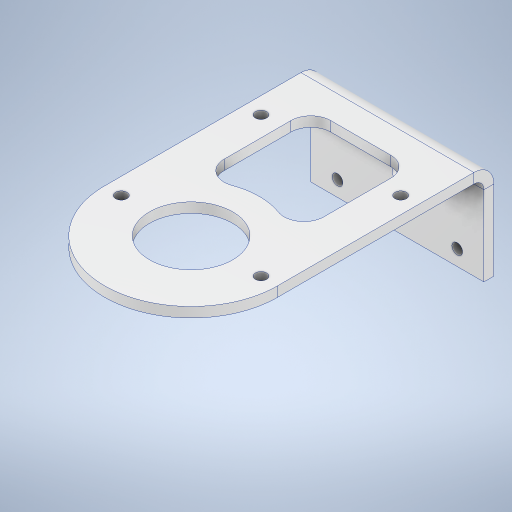
# Autodesk Inventor part: toe_front
Saved by Autodesk Inventor 2024.1 (Build 281209000, 209)
## iProperties
Created: 2024-02-12
Part Number: toe_front
Material: アルミニウム 6061
Document SubType Name: Sheet Metal
Designer: hibik
Density: 2.7 g/cm^3
Sheet Metal Rule: Default_mm
Appearance: アルミニウム - フラット
Flat Pattern Width: 2.6 cm
Flat Pattern Length: 5.78929 cm
Flat Pattern Area: 15.0522 cm^2
Sheet Metal Width: 26.000 mm
Sheet Metal Length: 57.893 mm
Sheet Metal Area: 1505.216 mm^2
Author: hibik
Autodesk Inventor part; units mm, degrees
ref_plane "YZ Plane" through (0, 0, 0) normal (1, 0, 0) x (0, 1, 0)
ref_plane "XZ Plane" through (0, 0, 0) normal (0, 1, 0) x (-1, 0, 0)
ref_plane "XY Plane" through (0, 0, 0) normal (0, 0, 1) x (1, 0, 0)
sketch "スケッチ1" plane through (0, 0, 0) normal (0, 1, 0) x (-1, 0, 0)
  line L0 (26, 0) -> (0, 0)
  line L1 (0, 0) -> (0, -89.5474)
  line L2 (0, -89.5474) -> (26, -89.5474)
  line L3 (26, -89.5474) -> (26, 0)
  line L4 (26, 0) -> (0, 0)
  line L5 (0, 0) -> (0, 70)
  line L6 (0, 70) -> (26, 70)
  line L7 (26, 70) -> (26, 0)
  line L8 (26, 32.5) -> (0, 32.5)
  circle A0 centre (13, 32.5) radius 6.25
  circle A1 centre (13, 32.5) radius 13
  point P0 (26, 32.5)
  point P1 (0, 32.5)
  dimension "d2" = 70
  dimension "d3" = 26
  dimension "d4" = 32.5
  dimension "d5" = 12.5
  measures "d2" distance of L4.end L5.end
  measures "d3" distance of L5.end L6.end
  measures "d4" distance between parallel lines of L0 L8
  measures "d5" diameter of A0
extrude "プレート1" add sketch "スケッチ1" along normal blind 1.5 contours L0 L5 A1 L7 | A1 L8 A0 | L8 A0 A1
sketch "スケッチ3" plane through (0, 1.5, 0) normal (0, 1, 0) x (1, 0, 0)
  circle A0 centre (-23.5, -32.5) radius 0.85 projected
  circle A1 centre (-23.5, -11.5) radius 0.85 projected
  circle A2 centre (-2.5, -11.5) radius 0.85 projected
  circle A3 centre (-2.5, -32.5) radius 0.85 projected
  point P0 (0, 0)
extrude "切り取り1" cut sketch "スケッチ3" against normal blind 1.5
sketch "スケッチ4" plane through (0, 1.5, 1.5) normal (0, 0, -1) x (-1, 0, 0)
  line L0 (26, 0) -> (0, 0)
  line L1 (0, 0) -> (0, -15)
  line L2 (0, -15) -> (26, -15)
  line L3 (26, -15) -> (26, 0)
  constraints: 6 end point, 1 horizontal, 1 perpendicular, 1 vertical
edge flange "フランジ2" height 15 angle 90 thickness 1.5 bend radius 1.5 thickness toward (0, 0, -1) relief straight relief width 1.5 relief depth 0.75 edges at (-13, 0, 0) wall of the first edge with corners at (-26, 1.5, 1.5) (0, 1.5, 1.5) (0, -13.5, 1.5) (-26, -13.5, 1.5)
bend "曲げ2"
corner "コーナー2"
sketch "スケッチ5" plane through (0, -13.5, 0) normal (0, 0, -1) x (-1, 0, 0)
  line L0 (0, 0) -> (26, 0)
  line L1 (26, 0) -> (26, 15)
  line L2 (26, 15) -> (0, 15)
  line L3 (0, 15) -> (0, 0)
  line L4 (26, 12) -> (26, 0) projected
  line L5 (0, 0) -> (0, 12) projected
  line L6 (0, 15) -> (26, 0)
  line L7 (26, 15) -> (0, 0)
  line L8 (4, 12.6923) -> (22, 12.6923)
  line L9 (22, 12.6923) -> (22, 2.3077)
  line L10 (22, 2.3077) -> (4, 2.3077)
  line L11 (4, 2.3077) -> (4, 12.6923)
  circle A0 centre (4, 12.6923) radius 0.8
  circle A1 centre (22, 12.6923) radius 0.8
  circle A2 centre (4, 2.3077) radius 0.8
  circle A3 centre (22, 2.3077) radius 0.8
  circle A4 centre (13, 7.5) radius 0.8
  point P0 (0, 13.5)
  dimension "d35" = 15
  dimension "d36" = 4
  dimension "d37" = 1.6
  dimension "d38" = 1.6
  dimension "d39" = 1.6
  dimension "d40" = 1.6
  dimension "d43" = 1.6
  constraints: 20 end point, 5 centre point, 4 coincident, 4 parallel, 3 point on line, 2 collinear, 2 horizontal, 2 perpendicular, 1 midpoint
  measures "d35" distance between parallel lines of L0 L2
  measures "d36" distance between parallel lines of L3 L11
  measures "d37" diameter of A0
  measures "d38" diameter of A1
  measures "d39" diameter of A2
  measures "d40" diameter of A3
  measures "d43" diameter of A4
extrude "切り取り3" cut sketch "スケッチ5" against normal blind 1.5 contours A2 L11 L7 | L7 L10 A2 | A3 L10 L6 | L6 L9 A3 | L11 A2 L7 | L7 A2 L10 | L10 A3 L6 | L6 A3 L9 | A4 L6 L7 | L7 L6 A4 | L6 L7 A4 | L6 A4 L7
sketch "スケッチ6" plane through (0, 1.5, 0) normal (0, 1, 0) x (1, 0, 0)
  circle A0 centre (-2.5, -32.5) radius 0.85 projected
  circle A1 centre (-23.5, -32.5) radius 0.85 projected
  circle A2 centre (-23.5, -11.5) radius 0.85 projected
  circle A3 centre (-2.5, -11.5) radius 0.85 projected
  line L0 (-2.5, -32.5) -> (-23.5, -32.5)
  line L1 (-23.5, -32.5) -> (-23.5, -11.5)
  line L2 (-23.5, -11.5) -> (-2.5, -11.5)
  line L3 (-2.5, -11.5) -> (-2.5, -32.5)
  line L4 (-5.5, -32.5) -> (-20.5, -32.5)
  line L5 (-20.5, -20.0376) -> (-20.5, -10)
  line L6 (-17.5, -7) -> (-8.5, -7)
  line L7 (-5.5, -10) -> (-5.5, -20.0376)
  circle A4 centre (-13, -32.5) radius 6.25 projected
  line L8 (0, -3) -> (-26, -3) projected
  arc A5 (-9.5189, -22.8592) -> (-16.4811, -22.8592) centre (-13, -32.5) ccw
  arc A6 (-23.2186, -31.6979) -> (-23.2186, -33.3021) centre (-13, -32.5) ccw
  arc A7 (-2.7814, -33.3021) -> (-2.7814, -31.6979) centre (-13, -32.5) ccw
  arc A8 (-9.5189, -22.8592) -> (-5.5, -20.0376) centre (-8.5, -20.0376) ccw
  arc A9 (-20.5, -20.0376) -> (-16.4811, -22.8592) centre (-17.5, -20.0376) ccw
  arc A10 (-5.5, -10) -> (-8.5, -7) centre (-8.5, -10) ccw
  arc A11 (-17.5, -7) -> (-20.5, -10) centre (-17.5, -10) ccw
  point P0 (0, 0)
  point P1 (-20.5, -7)
  point P2 (-5.5, -7)
  point P3 (-5.5, -25.5134)
  point P4 (-20.5, -25.5134)
  dimension "d46" = 3
  dimension "d47" = 3
  dimension "d49" = 4
  dimension "d50" = 4
  dimension "d53" = 3
  dimension "d54" = 3
  constraints: 20 point on circle, 16 end point, 8 tangent, 7 centre point, 7 point on line, 4 parallel, 2 equal radius, 2 horizontal, 2 perpendicular, 1 concentric, 1 midpoint
  measures "d46" distance between parallel lines of L3 L7
  measures "d47" distance between parallel lines of L1 L5
  measures "d49" distance between parallel lines of L8 L6
  measures "d50" radial gap between concentric circles of A4 A5
  measures "d53" radius of A8
  measures "d54" radius of A9
extrude "切り取り4" cut sketch "スケッチ6" against normal blind 1.5 contours L7 A8 A5 A9 L5 L2 | L2 L5 A11 L6 A10 L7
equation "\"d23\" = Thickness"
equation "\"d44\" = Thickness"
equation "\"d51\" = Thickness"
equation "\"d12\" = Thickness"
equation "\"d25\" = BendReliefWidth"
equation "\"d26\" = BendReliefDepth"
equation "\"d27\" = MinimumRemnant"
equation "\"d28\" = TransitionRadius"
equation "\"d31\" = BendRadius"
equation "\"d32\" = CornerReliefSize"
equation "\"d33\" = GapSize"
equation "\"d34\" = JacobiRadiusSize"
equation "\"BendRadius\" = Thickness"
equation "\"BendReliefWidth\" = Thickness"
equation "\"BendReliefDepth\" = 0.5 * Thickness"
equation "\"CornerReliefSize\" = 4 * Thickness"
equation "\"MinimumRemnant\" = 2 * Thickness"
equation "\"TransitionRadius\" = BendRadius"
equation "\"JacobiRadiusSize\" = BendRadius"
equation "\"GapSize\" = Thickness"
equation "\"Thickness\" = 1.5"
